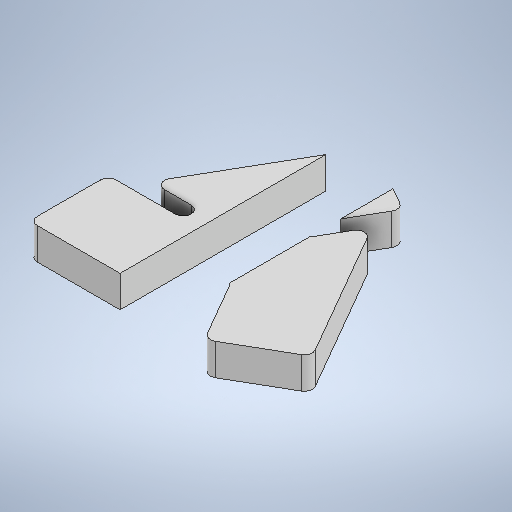
# Autodesk Inventor part: RT_FRM_MC_008_TopPlate_Support
Saved by Autodesk Inventor 2025.4 (Build 294407000, 407)
## iProperties
Created: 2026-04-28
Part Number: RT_FRM_MC_008_TopPlate_Support
Material: Generic
Document SubType Name: Modeling
Designer: louis
Density: 1 g/cm^3
Appearance: Default
Author: louis
Autodesk Inventor part; units mm, degrees
ref_plane "YZ Plane" through (0, 0, 0) normal (1, 0, 0) x (0, 1, 0)
ref_plane "XZ Plane" through (0, 0, 0) normal (0, 1, 0) x (-1, 0, 0)
ref_plane "XY Plane" through (0, 0, 0) normal (0, 0, 1) x (1, 0, 0)
sketch "Sketch1" plane through (0, 0, 0) normal (0, 1, 0) x (-1, 0, 0)
  line L0 (25, -2.5) -> (135, -2.5)
  line L1 (135, 0) -> (25, 0)
  line L2 (0, 0) -> (25, 0)
  circle A0 centre (0, 0) radius 200 construction
  line L3 (50, 0) -> (103.8137, 0) construction
  line L4 (130, 26.5) -> (30, 26.5)
  line L5 (30, 26.5) -> (30, 76.5)
  line L6 (30, 76.5) -> (130, 76.5)
  line L7 (130, 76.5) -> (130, 26.5)
  line L8 (80, 26.5) -> (80, 0) construction
  line L9 (80, 76.5) -> (80, 26.5) construction
  line L10 (121, 40.5) -> (80, 40.5) construction
  line L11 (121, 40.5) -> (121, 67) construction
  line L12 (199.7498, -10) -> (60, -10)
  line L13 (60, -10) -> (60, 10)
  line L14 (60, 10) -> (199.7498, 10)
  line L15 (199.7498, 10) -> (199.7498, -10)
  line L16 (0, 0) -> (0, 200)
  line L17 (155, 10) -> (155, 110)
  line L18 (155, 110) -> (-63.5085, 110)
  line L19 (-63.5085, 110) -> (0, 0)
  circle A1 centre (0, 0) radius 300 construction
  line L20 (-300, -380) -> (-300, -300) construction
  line L21 (-300, -300) -> (-380, -300) construction
  line L22 (-380, -300) -> (-380, -380) construction
  line L23 (-380, -380) -> (-300, -380) construction
  line L24 (-300, -380) -> (-380, -300) construction
  line L25 (-300, -300) -> (-380, -380) construction
  line L26 (-300, 300) -> (-300, 380) construction
  line L27 (-300, 380) -> (-380, 380) construction
  line L28 (-380, 380) -> (-380, 300) construction
  line L29 (-380, 300) -> (-300, 300) construction
  line L30 (-300, 300) -> (-380, 380) construction
  line L31 (-300, 380) -> (-380, 300) construction
  line L32 (380, 300) -> (380, 380) construction
  line L33 (380, 380) -> (300, 380) construction
  line L34 (300, 380) -> (300, 300) construction
  line L35 (300, 300) -> (380, 300) construction
  line L36 (380, 300) -> (300, 380) construction
  line L37 (380, 380) -> (300, 300) construction
  line L38 (380, -380) -> (380, -300) construction
  line L39 (380, -300) -> (300, -300) construction
  line L40 (300, -300) -> (300, -380) construction
  line L41 (300, -380) -> (380, -380) construction
  line L42 (380, -380) -> (300, -300) construction
  line L43 (380, -300) -> (300, -380) construction
  line L44 (300, -300) -> (300, 300) construction
  line L45 (300, 300) -> (-300, 300) construction
  line L46 (-300, 300) -> (-300, -300) construction
  line L47 (-300, -300) -> (300, -300) construction
  point P0 (39, 40.5)
  point P1 (39, 67)
  point P2 (190.7878, -60)
  point P3 (60, 0)
  dimension "d0" = 110
  dimension "d2" = 2.5
  dimension "d4" = 80
  dimension "d9" = 400
  dimension "d11" = 29
  dimension "d12" = 50
  dimension "d13" = 100
  dimension "d14" = 26.5
  dimension "d15" = 82
  dimension "d26" = 20
  dimension "d27" = 20
  dimension "d33" = 9.5
  dimension "d40" = 50
  dimension "d46" = 120
  dimension "d47" = 100
  dimension "d48" = 25
  dimension "d74" = 80
  dimension "d75" = 80
  dimension "d78" = 80
  dimension "d79" = 80
  dimension "d80" = 80
  dimension "d81" = 80
  dimension "d82" = 80
  dimension "d83" = 80
  dimension "d84" = 600
  constraints: 96 end point, 14 perpendicular, 12 parallel, 7 vertical, 4 horizontal, 4 point on circle, 3 coincident, 3 midpoint, 3 point on line, 3 tangent, 2 centre point, 2 symmetric about line, 1 collinear
  measures "d0" distance of L0.end L0.start
  measures "d2" distance between parallel lines of L0 L1
  measures "d4" distance of L2.start L8.end
  measures "d9" diameter of A0
  measures "d11" distance from line of L0 L4.start
  measures "d12" distance of L6.end L4.start
  measures "d13" distance of L4.start L4.end
  measures "d14" distance of L11.end L10.start
  measures "d15" distance of L10.start point (39, 40.5)
  measures "d26" distance between parallel lines of L14 L12
  measures "d27" distance between parallel lines of L8 L13
  measures "d33" distance from line of L6 L11.end
  measures "d40" distance from line of L12 point (190.788, -60)
  measures "d46" angle of L19 L2
  measures "d47" distance of L17.start L17.end
  measures "d48" distance between parallel lines of L17 L7
  measures "d74" distance of L21.end L22.end
  measures "d75" distance of L22.end L20.start
  measures "d78" distance of L27.end L28.end
  measures "d79" distance of L28.end L26.start
  measures "d80" distance of L33.end L34.end
  measures "d81" distance of L34.end L32.start
  measures "d82" distance of L39.end L40.end
  measures "d83" distance of L40.end L38.start
  measures "d84" diameter of A1
extrude "Extrusion1" add sketch "Sketch1" against normal blind 10 contours L1 L2 L16 L18 L17 L14 L13 | L19 L18 L16 | L4 L5 L6 L7
pattern_circular "Circular Pattern2" count 3 over 360 about axis through (0, 0, 0) along (0, -1, 0) of "Extrusion1"
hole "Hole1" at (-121, 0, 40.5) at (-39, 0, 40.5) at (-121, 0, 67) at (-39, 0, 67) direction (0, -1, 0) diameter 5.5 end through all counterbore diameter 10 counterbore depth 5 clearance for "Socket Head Cap Screw" size "M5" standard "Ansi Metric M Profile"
extrude "Extrusion2" cut sketch "Sketch1" against normal blind 10 contours L13 L14 L15 L12
pattern_circular "Circular Pattern1" count 3 over 360 about axis through (0, -10, 0) along (0, 1, 0) of "Hole1", "Extrusion2"
fillet "Fillet1" radius 10 15 edges at (21.3397, -5, 56.9615) (38.6603, -5, -46.9615) (-60, -5, -10) (-60, -5, 10) (38.6603, -5, 46.9615) (21.3397, -5, -56.9615) (-155, -5, 110) (-155, -5, 10) (51.9615, -5, 110) (86.1603, -5, 129.2339) (172.7628, -5, 79.2339) (69.282, -5, -100) (68.8397, -5, -139.2339) (-17.7628, -5, -189.2339) (-121.2436, -5, -10)
sketch "Sketch2" plane through (0, -10, 0) normal (0, 1, 0) x (1, 0, 0)
  line L0 (-70, 0) -> (0, 0) construction
  line L1 (0, 0) -> (0, 200) construction
  line L2 (-20, 0) -> (-20, 20) construction
  line L3 (-20, 20) -> (20, 20) construction
  line L4 (20, 20) -> (20, 0) construction
  line L5 (20, 0) -> (-20, 0) construction
  arc A0 (-70, -10) -> (-70, 10) centre (-70, 0) ccw projected
  line L6 (-20, -20) -> (-20, -100) construction
  line L7 (-20, -100) -> (20, -100) construction
  line L8 (20, 0) -> (20, -102.2687) construction
  point P0 (-20, 150)
  point P1 (20, 150)
  point P2 (-60, 0)
  point P3 (20, -20)
  dimension "d52" = 90
  dimension "d53" = 200
  dimension "d54" = 40
  dimension "d55" = 20
  dimension "d58" = 130
  dimension "d85" = 80
  constraints: 18 end point, 5 perpendicular, 3 coincident, 3 symmetric about line, 2 point on line, 2 vertical, 1 horizontal, 1 parallel, 2 other
  measures "d52" angle of L0 L1
  measures "d53" distance of L0.end L1.end
  measures "d54" distance of L4.end L2.start
  measures "d55" distance of L3.end L4.end
  measures "d58" distance of point (-20, 20) point (-20, 150)
  measures "d85" distance of L6.start L6.end
hole "Hole2" at (20, -10, -20) at (-20, -10, -20) at (-20, -10, -150) at (20, -10, -150) at (-20, -10, 100) at (20, -10, 100) at (20, -10, 20) at (-20, -10, 20) direction (0, 1, 0) diameter 5.5 end through all counterbore diameter 10 counterbore depth 5 clearance for "Socket Head Cap Screw" size "M5" standard "Ansi Metric M Profile"
sketch "Sketch3" plane through (0, 0, 0) normal (0, 1, 0) x (1, 0, 0)
  circle A0 centre (-20, -20) radius 2.75 projected
  circle A1 centre (20, -20) radius 2.75 projected
  circle A2 centre (20, -100) radius 2.75 projected
  circle A3 centre (-20, -100) radius 2.75 projected
  circle A4 centre (20, 150) radius 2.75 projected
  circle A5 centre (-20, 150) radius 2.75 projected
  circle A6 centre (-20, 20) radius 2.75 projected
  circle A7 centre (20, 20) radius 2.75 projected
  circle A8 centre (-39, -67) radius 5 projected
  circle A9 centre (-121, -67) radius 5 projected
  circle A10 centre (-39, -40.5) radius 5 projected
  circle A11 centre (-121, -40.5) radius 5 projected
  circle A12 centre (77.5237, -0.275) radius 5 projected
  circle A13 centre (95.574, -84.5391) radius 5 projected
  circle A14 centre (54.574, -13.525) radius 5 projected
  circle A15 centre (118.5237, -71.2891) radius 5 projected
  circle A16 centre (-38.5237, 67.275) radius 5 projected
  circle A17 centre (25.426, 125.0391) radius 5 projected
  circle A18 centre (-15.574, 54.025) radius 5 projected
  circle A19 centre (2.4763, 138.2891) radius 5 projected
  arc A20 (-112.5833, 25) -> (-103.923, 10) centre (-103.923, 20) ccw projected
  line L0 (-103.923, 10) -> (-70, 10) projected
  arc A21 (-70, -10) -> (-70, 10) centre (-70, 0) ccw projected
  line L1 (-70, -10) -> (-145, -10) projected
  arc A22 (-145, -10) -> (-155, -20) centre (-145, -20) ccw projected
  line L2 (-155, -20) -> (-155, -100) projected
  arc A23 (-155, -100) -> (-145, -110) centre (-145, -100) ccw projected
  line L3 (-145, -110) -> (34.641, -110) projected
  arc A24 (34.641, -110) -> (43.3013, -95) centre (34.641, -100) ccw projected
  line L4 (43.3013, -95) -> (26.3397, -65.6218) projected
  arc A25 (43.6603, -55.6218) -> (26.3397, -65.6218) centre (35, -60.6218) ccw projected
  line L5 (43.6603, -55.6218) -> (81.1603, -120.5737) projected
  arc A26 (81.1603, -120.5737) -> (94.8205, -124.2339) centre (89.8205, -115.5737) ccw projected
  line L6 (94.8205, -124.2339) -> (164.1025, -84.2339) projected
  arc A27 (164.1025, -84.2339) -> (167.7628, -70.5737) centre (159.1025, -75.5737) ccw projected
  line L7 (167.7628, -70.5737) -> (77.9423, 85) projected
  arc A28 (77.9423, 85) -> (60.6218, 85) centre (69.282, 80) ccw projected
  line L8 (60.6218, 85) -> (43.6603, 55.6218) projected
  arc A29 (26.3397, 65.6218) -> (43.6603, 55.6218) centre (35, 60.6218) ccw projected
  line L9 (26.3397, 65.6218) -> (63.8397, 130.5737) projected
  arc A30 (63.8397, 130.5737) -> (60.1795, 144.2339) centre (55.1795, 135.5737) ccw projected
  line L10 (60.1795, 144.2339) -> (-9.1025, 184.2339) projected
  arc A31 (-9.1025, 184.2339) -> (-22.7628, 180.5737) centre (-14.1025, 175.5737) ccw projected
  line L11 (-22.7628, 180.5737) -> (-112.5833, 25) projected
  line L12 (-40, 185.5737) -> (40, 185.5737)
  line L13 (40, 185.5737) -> (40, -110)
  line L14 (40, -110) -> (-40, -110)
  line L15 (-40, -110) -> (-40, 185.5737)
  arc A32 (34.641, -110) -> (43.3013, -95) centre (34.641, -100) ccw projected
  circle A33 centre (-20, 20) radius 5 construction
  line L16 (-20, 20) -> (20, -20) construction
  line L17 (0, 0) -> (40, 0) construction
  point P0 (40, 155.8846)
  point P1 (40, 89.282)
  point P2 (40, 51.9615)
  point P3 (40, -51.9615)
  point P4 (-40, 150.718)
  dimension "d86" = 80
  dimension "d87" = 40
  constraints: 12 end point, 2 parallel, 2 perpendicular, 2 tangent, 1 horizontal, 1 point on line
  measures "d86" distance of L13.end L14.end
  measures "d87" distance of L17.start L17.end
extrude "Extrusion3" add sketch "Sketch3" along normal blind 40 separate body contours L15 A8 | A8 L15 L3 A23 L2 A22 L1 A21 L0 A20 L11 A16 A10 | A10 L15 | A16 L15 | L13 A29 L8 A28 L7 A27 L6 A26 L5 A25 | L13 L10 A30 L9 | A9 | A11 | A12 | A13 | A14 | A15 picked at (-42.1524, -65.8032) picked at (-41.3204, -40.293) picked at (-41.1635, 67.4672)
body "Solid1"
body "Solid2"
